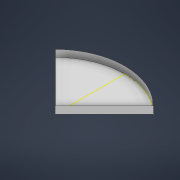
# Autodesk Inventor part: 棒球底座
Saved by Autodesk Inventor 2021 (Build 250183000, 183)
## iProperties
Created: 2020-12-20
Part Number: 棒球底座
Material: 一般
Document SubType Name: Modeling
Designer: zihon
Density: 1 g/cm^3
Appearance: 預設
Author: zihon
Autodesk Inventor part; units mm, degrees
ref_plane "YZ Plane" through (0, 0, 0) normal (1, 0, 0) x (0, 1, 0)
ref_plane "XZ Plane" through (0, 0, 0) normal (0, 1, 0) x (-1, 0, 0)
ref_plane "XY Plane" through (0, 0, 0) normal (0, 0, 1) x (1, 0, 0)
sketch "草圖1" plane through (0, 0, 0) normal (0, 1, 0) x (-1, 0, 0)
  line L0 (0, 0) -> (-1060.6602, -1060.6602)
  arc A0 (-1060.6602, -1060.6602) -> (0, -1500) centre (0, 0) ccw
  line L1 (0, -1935.3977) -> (0, 330.8159) projected
  arc A1 (-1067.7254, -1060.6543) -> (0, -1505) centre (0, 0) ccw
  line L2 (-1067.7254, -1060.6543) -> (0, 7.0711)
  line L3 (0, 0) -> (1060.6602, -1060.6602)
  arc A2 (0, -1500) -> (1060.6602, -1060.6602) centre (0, 0) ccw
  arc A3 (0, -1505) -> (1067.7254, -1060.6543) centre (0, 0) ccw
  line L4 (1067.7254, -1060.6543) -> (0, 7.0711)
  dimension "d0" = 45
  dimension "d2" = 1500
  dimension "d3" = 5
  dimension "d5" = 5
  constraints: 8 end point, 8 point on circle, 4 centre point, 2 coincident, 2 point on line, 2 symmetric about line, 1 parallel, 2 other
  measures "d0" angle of L1 L0
  measures "d2" distance of L0.start L0.end
  measures "d3" radial gap between concentric circles of A0 A1
  measures "d5" distance between parallel lines of L0 L2
extrude "擠出1" add sketch "草圖1" against normal blind 5 contours L1 A0 L0 | L0 A0 L1 A1 L2
extrude "擠出6" add sketch "草圖1" along normal blind 150 contours L0 A0 L1 A1 L2
sketch "草圖29" plane through (0, 0, 0) normal (0, 1, 0) x (1, 0, 0)
  line L0 (0, 0) -> (1060.6602, 1060.6602) projected
  arc A0 (1060.6602, 1060.6602) -> (0, 1500) centre (0, 0) ccw projected
  line L1 (0, 1500) -> (0, 0) projected
mirror "鏡射6" about plane through (0, 0, 0) normal (1, 0, 0) of "擠出1", "擠出6"
